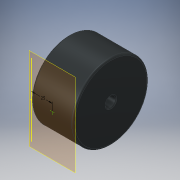
# Autodesk Inventor part: ciezarek
Saved by Autodesk Inventor 2019 (Build 230136000, 136)
## iProperties
Created: 2020-08-31
Part Number: ciezarek
Material: Iron, Cast
Document SubType Name: Modeling
Designer: estee
Density: 7.15 g/cm^3
Appearance: Iron Gray
Author: estee
Autodesk Inventor part; units mm, degrees
ref_plane "YZ Plane" through (0, 0, 0) normal (1, 0, 0) x (0, 1, 0)
ref_plane "XZ Plane" through (0, 0, 0) normal (0, 1, 0) x (-1, 0, 0)
sketch "Sketch1" plane through (0, 0, 0) normal (1, 0, 0) x (0, 1, 0)
  circle A0 centre (0, 0) radius 45
  circle A1 centre (0, 0) radius 6.1
  dimension "d0" = 90
  dimension "d1" = 12.2
  constraints: 2 centre point, 2 coincident
  measures "d0" diameter of A0
  measures "d1" diameter of A1
extrude "Extrusion1" add sketch "Sketch1" along normal blind 50
chamfer "Chamfer1" distance 1 angle 45 2 edges at (50, -6.1, 0) (0, -6.1, 0)
fillet "Fillet1" radius 2 2 edges at (0, -45, 0) (50, -45, 0)
ref_plane "Work Plane1" through (0, 0, 45) normal (0, 0, 1) x (1, 0, 0)
sketch "Sketch2" plane through (0, 0, 45) normal (0, 0, 1) x (1, 0, 0)
  line L0 (0, -43) -> (0, 43) projected
  point P0 (0, 0)
  point P1 (25, 0)
  dimension "d9" = 25
  measures "d9" distance from line of L0 point (25, 0)
body "Solid1"
